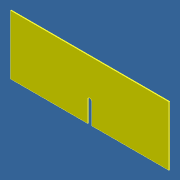
# Autodesk Inventor part: FE-00015
Saved by Autodesk Inventor 2012 (Build 160160000, 160)
## iProperties
Created: 2009-01-02
Part Number: FE-00015
Document SubType Name: Modeling
Designer: dfoster
Density: 1 g/cm^3
Material: Default
Author: dfoster
Autodesk Inventor part; units mm, degrees
ref_plane "YZ Plane" through (0, 0, 0) normal (1, 0, 0) x (0, 1, 0)
ref_plane "XZ Plane" through (0, 0, 0) normal (0, 1, 0) x (-1, 0, 0)
ref_plane "XY Plane" through (0, 0, 0) normal (0, 0, 1) x (1, 0, 0)
sketch "Sketch1" plane through (0, 0, 0) normal (0, 0, 1) x (1, 0, 0)
  line L0 (-27.0845, 23.2922) -> (582.5155, 23.2922)
  line L1 (582.5155, 23.2922) -> (582.5155, -205.3078)
  line L2 (-27.0845, -205.3078) -> (-27.0845, 23.2922)
  line L3 (269.778, -205.3078) -> (269.778, -124.3453)
  line L4 (285.653, -124.3453) -> (285.653, -205.3078)
  arc A0 (285.653, -124.3453) -> (269.778, -124.3453) centre (277.7155, -124.3453) ccw
  line L5 (582.5155, -205.3078) -> (285.653, -205.3078)
  line L6 (269.778, -205.3078) -> (-27.0845, -205.3078)
  dimension "d0" = 609.6
  dimension "d1" = 228.6
  dimension "d2" = 15.875
  dimension "d3" = 304.8
  dimension "d4" = 80.9625
  constraints: 14 end point, 4 parallel, 3 perpendicular, 2 point on circle, 2 tangent, 1 centre point, 1 collinear, 1 horizontal
  measures "d0" distance of L0.start L0.end
  measures "d1" distance of L2.start L0.start
  measures "d2" distance between parallel lines of L4 L3
  measures "d3" distance from line of A0.centre L2
  measures "d4" distance from line of A0.centre L6
extrude "Extrusion1" add sketch "Sketch1" along normal blind 3.175
body "Solid1"
